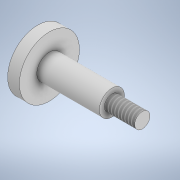
# Autodesk Inventor part: Pancake Shifter Shaft
Saved by Autodesk Inventor 2021 (Build 250183000, 183)
## iProperties
Created: 2021-02-24
Part Number: Pancake Shifter Shaft
Material: Generic
Document SubType Name: Modeling
Designer: aidan
Density: 1 g/cm^3
Appearance: Default
Author: aidan
Autodesk Inventor part; units mm, degrees
ref_plane "YZ Plane" through (0, 0, 0) normal (1, 0, 0) x (0, 1, 0)
ref_plane "XZ Plane" through (0, 0, 0) normal (0, 1, 0) x (-1, 0, 0)
ref_plane "XY Plane" through (0, 0, 0) normal (0, 0, 1) x (1, 0, 0)
sketch "Sketch1" plane through (0, 0, 0) normal (0, 0, 1) x (1, 0, 0)
  line L0 (0, 0) -> (0, 9.525)
  line L1 (0, 9.525) -> (3.7084, 9.525)
  line L2 (3.7084, 9.525) -> (3.7084, 3.9751)
  line L3 (3.7084, 3.9751) -> (23.5458, 3.9751)
  line L4 (23.5458, 3.9751) -> (23.5458, 2.413)
  line L5 (23.5458, 2.413) -> (33.1978, 2.413)
  line L6 (33.1978, 2.413) -> (33.1978, 0)
  line L7 (33.1978, 0) -> (0, 0)
  dimension "d0" = 9.525
  dimension "d1" = 3.9751
  dimension "d2" = 3.7084
  dimension "d3" = 9.652
  dimension "d4" = 33.1978
  dimension "d5" = 2.413
  constraints: 16 end point, 7 perpendicular, 1 vertical
  measures "d0" distance of L0.start L0.end
  measures "d1" distance between parallel lines of L7 L3
  measures "d2" distance of L0.end L1.end
  measures "d3" distance of L4.end L5.end
  measures "d4" distance from line of L6.end L0
  measures "d5" distance between parallel lines of L7 L5
revolve "Revolution1" add sketch "Sketch1" angle 360 about axis through (33.1978, 0, 0) along (-1, 0, 0)
thread "Thread1" size "10-24 UNC" class "2A" standard "ANSI Unified Screw Threads" full length
body "Solid1"
